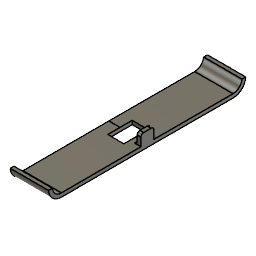
Tapa trasera intermedia 1-2 piso (Autodesk Fusion 360 design; units mm, degrees)
Autodesk Fusion 360 part; units mm, degrees
note: some values were not read from the file. Chosen so that the rebuilt part matches the saved one: which pieces of a blend or face edit are solid. Set by a fixed rule: which sketch regions a step uses.
sketch "Boceto1" plane through (0, 0, 0) normal (1, 0, 0) x (0, 0, -1)
  line L0 (-66.6474, -134.8235) -> (0.3307, -134.702)
  arc A0 (67.3089, -134.8235) -> (77.3307, -124.8933) centre (67.327, -124.8196) ccw
  line L1 (67.3089, -134.8235) -> (0.3307, -134.702)
  arc A1 (-76.6693, -124.8933) -> (-66.6474, -134.8235) centre (-66.6656, -124.8196) ccw
  arc A2 (-73.6692, -124.8933) -> (-66.6529, -131.8235) centre (-66.6656, -124.8196) ccw
  line L2 (-66.6529, -131.8235) -> (0.3307, -131.702)
  line L3 (67.3143, -131.8235) -> (0.3307, -131.702)
  arc A3 (67.3143, -131.8235) -> (74.3306, -124.8933) centre (67.327, -124.8196) ccw
  line L4 (-76.6693, -124.8933) -> (-73.6692, -124.8933)
  line L5 (77.3307, -124.8933) -> (74.3306, -124.8933)
  constraint tangent L0 A1
  constraint horizontal L4
  constraint horizontal L5
  constraint concentric A1 A2
  constraint concentric A0 A3
extrude "Extruir1" add sketch "Boceto1" along normal blind 30 makes body 1
sketch "Boceto2" plane through (30, 0, 0) normal (1, 0, 0) x (0, 0, -1)
  arc A0 (67.3089, -134.8235) -> (77.3307, -124.8933) centre (67.327, -124.8196) ccw
  line L0 (77.3307, -124.8933) -> (74.3306, -124.8933)
  arc A1 (67.3143, -131.8235) -> (74.3306, -124.8933) centre (67.327, -124.8196) ccw
  line L1 (67.3143, -131.8235) -> (0.3307, -131.702)
  line L2 (0.3307, -131.702) -> (-66.6529, -131.8235)
  arc A2 (-73.6692, -124.8933) -> (-66.6529, -131.8235) centre (-66.6656, -124.8196) ccw
  line L3 (-73.6692, -124.8933) -> (-76.6693, -124.8933)
  arc A3 (-76.6693, -124.8933) -> (-66.6474, -134.8235) centre (-66.6656, -124.8196) ccw
  line L4 (-66.6474, -134.8235) -> (0.3307, -134.702)
  line L5 (0.3307, -134.702) -> (67.3089, -134.8235)
  line L6 (5.4259, -131.1368) -> (-4.5741, -131.1368)
  line L7 (-4.5741, -131.1368) -> (-4.5741, -123.1368)
  line L8 (-4.5741, -123.1368) -> (5.4259, -123.1368)
  line L9 (5.4259, -123.1368) -> (5.4259, -131.1368)
  dimension "d6" = 10
  dimension "d7" = 8
  dimension "d8" = 68.9047
  constraint horizontal L6
  constraint vertical L7
  constraint horizontal L8
  constraint vertical L9
  measures "d6" distance of L7.end L8.end
  measures "d7" distance of L6.end L7.end
  measures "d8" distance of L0.end L9
extrude "Extruir2" add sketch "Boceto2" against normal blind 3 separate body contours L6 L7 L8 L9 makes body 2
extrude "Extruir3" add 1 faces at (29, -131.1368, -2.0926) along direction (0, -1, 0) up to surface end surface through (0, -131.8235, -67.3143) normal (0, -0.999998, 0.001814) offset 0 on bodies 2 bodies 1 2
extrude "Extruir4" add 1 faces at (29, -131.6961, 2.9392) along direction (0, -0.999998, 0.001814) up to surface end surface through (0, -131.8235, 66.6529) normal (0, 0.999998, 0.001814) offset 0 on bodies 1 bodies 1
fillet "Empalme1" radius 2 2 edges at (28.5, -123.1368, -5.4259) (28.5, -123.1368, 4.5741) on bodies 1
fillet "Empalme2" radius 2 2 edges at (27, -131.7065, 2.1217) (27, -131.7066, -2.8783) on bodies 1
sketch "Boceto3" plane through (0, -134.7022, -0.2444) normal (0, -0.999998, -0.001814) x (-1, 0, 0)
  line L0 (0, -66.8919) -> (0, 0.0863)
  line L1 (0, 0.0863) -> (-30, 0.0863)
  line L2 (-30, 0.0863) -> (-30, -66.8919)
  line L3 (-30, -66.8919) -> (0, -66.8919)
  line L4 (-21.25, -9.4137) -> (-8.75, -9.4137)
  line L5 (-8.75, -9.4137) -> (-8.75, 9.5863)
  line L6 (-8.75, 9.5863) -> (-21.25, 9.5863)
  line L7 (-21.25, 9.5863) -> (-21.25, -9.4137)
  line L8 (-21.25, -9.4137) -> (-8.75, 9.5863) construction
  line L9 (-8.75, -9.4137) -> (-21.25, 9.5863) construction
  point P0 (-15, 0.0863)
  dimension "d19" = 19
  dimension "d20" = 12.5
  constraint horizontal L4
  constraint perpendicular L4 L5
  constraint parallel L4 L6
  constraint parallel L5 L7
  constraint coincident L8 P0
  constraint coincident L9 P0
  constraint midpoint L1 P0
  measures "d19" distance of L4.end L5.end
  measures "d20" distance of L4.start L4.end
extrude "Extruir5" cut sketch "Boceto3" against normal through all contours L1 L4 L5 L7 | L1 L5 L6 L7 bodies 1
extrude "Extruir6" cut sketch "Boceto3" along normal through all contours L1 L5 L6 L7 bodies 1
sketch "Boceto4" plane through (30, 0, 0) normal (1, 0, 0) x (0, 0, -1)
  line L0 (77.3307, -124.8933) -> (74.3306, -124.8933)
  line L1 (73.3903, -125.4743) -> (77.3307, -125.4743)
  line L2 (77.3307, -125.4743) -> (77.3307, -124.8933)
  line L3 (77.3307, -124.8933) -> (73.3903, -124.8933)
  line L4 (73.3903, -124.8933) -> (73.3903, -125.4743)
  line L5 (-76.6693, -124.8933) -> (-73.6692, -124.8933)
  line L6 (-73.4648, -124.8933) -> (-77.1539, -124.8933)
  line L7 (-77.1539, -124.8933) -> (-77.1539, -125.2023)
  line L8 (-77.1539, -125.2023) -> (-73.4648, -125.2023)
  line L9 (-73.4648, -124.8933) -> (-73.4648, -125.2023)
  dimension "d23" = 0.581
  dimension "d24" = 0.309
  constraint horizontal L1
  constraint vertical L2
  constraint horizontal L3
  constraint vertical L4
  constraint coincident L0.start L2.end
  constraint horizontal L6
  constraint vertical L7
  constraint horizontal L8
  constraint vertical L9
  measures "d23" distance of L1 L3
  measures "d24" distance of L6 L8
extrude "Extruir7" cut sketch "Boceto4" against normal through all bodies 1
